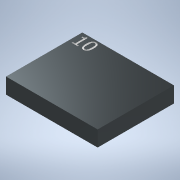
# Autodesk Inventor part: 10gram weight
Saved by Autodesk Inventor 2022 (Build 260153000, 153)
## iProperties
Created: 2021-08-25
Part Number: 10gram weight
Material: Generic
Document SubType Name: Modeling
Designer: benka
Density: 1 g/cm^3
Appearance: Default
Author: benka
Autodesk Inventor part; units mm, degrees
note: some values were not read from the file. Chosen so that the rebuilt part matches the saved one: direction of "Emboss1".
ref_plane "YZ Plane" through (0, 0, 0) normal (1, 0, 0) x (0, 1, 0)
ref_plane "XZ Plane" through (0, 0, 0) normal (0, 1, 0) x (-1, 0, 0)
ref_plane "XY Plane" through (0, 0, 0) normal (0, 0, 1) x (1, 0, 0)
sketch "Sketch1" plane through (0, 0, 0) normal (0, 1, 0) x (-1, 0, 0)
  line L0 (11.4, -9.5) -> (-11.4, -9.5)
  line L1 (-11.4, -9.5) -> (-11.4, 9.5)
  line L2 (-11.4, 9.5) -> (11.4, 9.5)
  line L3 (11.4, 9.5) -> (11.4, -9.5)
  point P0 (0, 0)
  point P1 (0, 0)
  dimension "d0" = 22.8
  dimension "d1" = 19
  constraints: 8 end point, 2 parallel, 1 horizontal, 1 perpendicular
  measures "d0" distance of L1.end L2.end
  measures "d1" distance of L0.end L1.end
extrude "Extrusion1" add sketch "Sketch1" along normal blind 3.9
sketch "Sketch2" plane through (0, 3.9, 0) normal (0, 1, 0) x (1, 0, 0)
  line L0 (-10.9508, 9.0636) -> (-5.7361, 9.0636) construction
  line L1 (-5.7361, 9.0636) -> (-5.7361, 4.6932) construction
  line L2 (-5.7361, 4.6932) -> (-10.9508, 4.6932) construction
  line L3 (-10.9508, 4.6932) -> (-10.9508, 9.0636) construction
  line L4 (-9.0019, 5.9538) -> (-10.4889, 5.9538)
  line L5 (-10.4889, 5.9538) -> (-10.4889, 6.265)
  line L6 (-10.4889, 6.265) -> (-9.9356, 6.265)
  line L7 (-9.9356, 6.265) -> (-9.9356, 8.3077)
  line L8 (-9.9356, 8.3077) -> (-10.4889, 8.3077)
  line L9 (-10.4889, 8.3077) -> (-10.4889, 8.5869)
  spline S0 degree 2 poles (-10.4889, 8.5869) (-10.1752, 8.5869) (-9.8788, 8.7647) (-9.859, 9.0117) knots 0 0 0 1 2 2 2
  line L10 (-9.859, 9.0117) -> (-9.5429, 9.0117)
  line L11 (-9.5429, 9.0117) -> (-9.5429, 6.265)
  line L12 (-9.5429, 6.265) -> (-9.0019, 6.265)
  line L13 (-9.0019, 6.265) -> (-9.0019, 5.9538)
  spline S1 degree 2 poles (-6.5443, 7.4778) (-6.5443, 6.6578) (-7.021, 5.8896) (-7.5175, 5.8896) knots 0 0 0 1 2 2 2
  spline S2 degree 2 poles (-7.5175, 5.8896) (-8.0213, 5.8896) (-8.4931, 6.6726) (-8.4931, 7.4754) knots 0 0 0 1 2 2 2
  spline S3 degree 2 poles (-8.4931, 7.4754) (-8.4931, 8.3003) (-8.0164, 9.0636) (-7.5175, 9.0636) knots 0 0 0 1 2 2 2
  spline S4 degree 2 poles (-7.5175, 9.0636) (-7.016, 9.0636) (-6.5443, 8.2732) (-6.5443, 7.4778) knots 0 0 0 1 2 2 2
  spline S5 degree 2 poles (-7.0679, 6.5491) (-7.0086, 6.6998) (-6.9592, 7.1641) (-6.9592, 7.4778) knots 0 0 0 1 2 2 2
  spline S6 degree 2 poles (-6.9592, 7.4778) (-6.9592, 7.7915) (-7.0086, 8.2534) (-7.0704, 8.409) knots 0 0 0 1 2 2 2
  spline S7 degree 2 poles (-7.0704, 8.409) (-7.1321, 8.5646) (-7.347, 8.7252) (-7.5175, 8.7252) knots 0 0 0 1 2 2 2
  spline S8 degree 2 poles (-7.5175, 8.7252) (-7.6879, 8.7252) (-7.9077, 8.5646) (-7.9719, 8.4041) knots 0 0 0 1 2 2 2
  spline S9 degree 2 poles (-7.9719, 8.4041) (-8.0337, 8.2485) (-8.0782, 7.7742) (-8.0782, 7.4754) knots 0 0 0 1 2 2 2
  spline S10 degree 2 poles (-8.0782, 7.4754) (-8.0782, 7.1543) (-8.0386, 6.7245) (-7.9744, 6.5565) knots 0 0 0 1 2 2 2
  spline S11 degree 2 poles (-7.9744, 6.5565) (-7.9151, 6.3984) (-7.6953, 6.228) (-7.5175, 6.228) knots 0 0 0 1 2 2 2
  spline S12 degree 2 poles (-7.5175, 6.228) (-7.3495, 6.228) (-7.1297, 6.3885) (-7.0679, 6.5491) knots 0 0 0 1 2 2 2
  point P0 (0, 0)
  constraints: 2 other
emboss "Emboss1" sketch "Sketch2" operation cut depth 0.3 direction (0, -1, 0)
body "Solid1"
